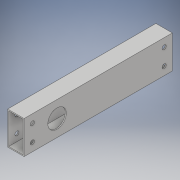
# Autodesk Inventor part: Roller Wheel Right Side Support Beam
Saved by Autodesk Inventor 2018 (Build 220112000, 112)
## iProperties
Created: 2020-02-25
Part Number: Roller Wheel Right Side Support Beam
Material: Generic
Document SubType Name: Modeling
Designer: T3500STATIC
Density: 1 g/cm^3
Appearance: Default
Author: T3500STATIC
Autodesk Inventor part; units mm, degrees
ref_plane "YZ Plane" through (0, 0, 0) normal (1, 0, 0) x (0, 1, 0)
ref_plane "XZ Plane" through (0, 0, 0) normal (0, 1, 0) x (-1, 0, 0)
ref_plane "XY Plane" through (0, 0, 0) normal (0, 0, 1) x (1, 0, 0)
sketch "Sketch1" plane through (0, 0, 0) normal (0, 0, 1) x (1, 0, 0)
  line L0 (0, 0) -> (25.4, 0)
  line L1 (25.4, 0) -> (25.4, 50.8)
  line L2 (25.4, 50.8) -> (0, 50.8)
  line L3 (0, 50.8) -> (0, 0)
  dimension "d0" = 25.4
  dimension "d1" = 50.8
  constraints: 8 end point, 2 parallel, 1 horizontal, 1 perpendicular
  measures "d0" distance of L2.end L1.end
  measures "d1" distance of L1.end L0.end
extrude "Extrusion1" add sketch "Sketch1" along normal blind 228.6
shell "Shell1" thickness 1.5875 removed faces 2 at (8.4667, 16.9333, 0) at (8.4667, 16.9333, 228.6)
hole "Hole3" at (25.4, 38.1, 12.7) direction (-1, 0, 0) diameter 6.35 end through all
hole "Hole4" at (25.4, 12.7, 12.7) direction (-1, 0, 0) diameter 6.35 end through all
hole "Hole5" at (25.4, 25.4, 177.8) direction (-1, 0, 0) diameter 28.575 end through all
hole "Hole7" at (25.4, 38.1, 215.9) direction (-1, 0, 0) diameter 6.35 end through all
hole "Hole8" at (25.4, 12.7, 215.9) direction (-1, 0, 0) diameter 6.35 end through all
body "Solid1"
